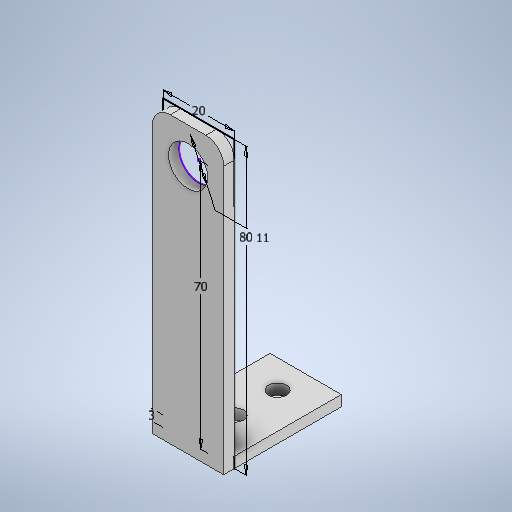
# Autodesk Inventor part: roll stand
Saved by Autodesk Inventor 2025.1 (Build 291241020, 241B)
## iProperties
Created: 2025-01-25
Part Number: roll stand
Material: Generic
Document SubType Name: Modeling
Designer: User
Density: 1 g/cm^3
Appearance: Default
Author: User
Autodesk Inventor part; units mm, degrees
ref_plane "YZ Plane" through (0, 0, 0) normal (1, 0, 0) x (0, 1, 0)
ref_plane "XZ Plane" through (0, 0, 0) normal (0, 1, 0) x (-1, 0, 0)
ref_plane "XY Plane" through (0, 0, 0) normal (0, 0, 1) x (1, 0, 0)
sketch "Sketch1" plane through (0, 0, 0) normal (0, 0, 1) x (1, 0, 0)
  line L0 (0, 0) -> (20, 0)
  line L1 (20, 0) -> (20, 80)
  line L2 (20, 80) -> (0, 80)
  line L3 (0, 80) -> (0, 0)
  circle A0 centre (10, 70) radius 5.5
  line L4 (20, 0) -> (0, 0)
  line L5 (0, 0) -> (0, 3)
  line L6 (0, 3) -> (20, 3)
  line L7 (20, 3) -> (20, 0)
  point P0 (10, 0)
  dimension "d0" = 20
  dimension "d1" = 80
  dimension "d2" = 11
  dimension "d3" = 70
  dimension "d7" = 3
  constraints: 16 end point, 4 parallel, 2 horizontal, 2 perpendicular, 1 centre point, 1 midpoint, 1 point on line
  measures "d0" distance of L2.end L1.end
  measures "d1" distance of L0.end L1.end
  measures "d2" diameter of A0
  measures "d3" distance of point (10, 0) A0.centre
  measures "d7" distance between parallel lines of L0 L6
extrude "Extrusion1" add sketch "Sketch1" along normal blind 3
fillet "Fillet1" radius 5 2 edges at (20, 80, 1.5) (0, 80, 1.5)
extrude "Extrusion2" add sketch "Sketch1" against normal blind 30 contours L3 L6 L1 L0
sketch "Sketch2" plane through (0, 3, 0) normal (0, 1, 0) x (1, 0, 0)
  circle A0 centre (10, 22.1006) radius 2.5
  circle A1 centre (10, 10.048) radius 2.5
  point P0 (0, 0)
  dimension "d10" = 5
  dimension "d11" = 5
  constraints: 2 centre point
  measures "d10" diameter of A0
  measures "d11" diameter of A1
extrude "Extrusion3" cut sketch "Sketch2" against normal through all
extrude "Extrusion4" cut sketch "Sketch1" along normal blind 10 contours A0
extrude "Extrusion5" cut sketch "Sketch1" along normal blind 10 contours A0
body "Solid1"
